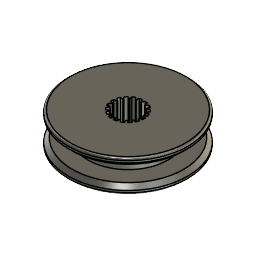
Spool60KGV0_v2 (Autodesk Fusion 360 design; units mm, degrees)
Autodesk Fusion 360 part; units mm, degrees
sketch "Sketch1" plane through (0, 0, 0) normal (0, 0, 1) x (1, 0, 0)
  line L0 (2.1718, 2.3549) -> (1.942, 2.5478)
  line L1 (2.1718, -2.3549) -> (2.7951, -2.7198)
  line L2 (-0.9579, 3.7805) -> (-0.9535, 3.0583)
  line L3 (1.942, -2.5478) -> (2.1718, -2.3549)
  line L4 (0.15, 3.2) -> (-0.15, 3.2)
  arc A0 (3.5568, -1.5998) -> (3.753, -1.0607) centre (0, 0) ccw
  line L5 (-0.15, 3.2) -> (-0.3929, 3.8802)
  arc A1 (3.753, 1.0607) -> (3.5568, 1.5998) centre (0, 0) ccw
  arc A2 (1.6963, -3.5118) -> (2.1931, -3.2249) centre (0, 0) ccw
  line L6 (2.7951, 2.7198) -> (2.1718, 2.3549)
  line L7 (-3.1253, -0.7034) -> (-3.753, -1.0607)
  arc A3 (-3.5568, 1.5998) -> (-3.753, 1.0607) centre (0, 0) ccw
  line L8 (-2.6963, 1.7299) -> (-2.8463, 1.4701)
  circle A4 centre (0, 0) radius 1.5
  line L9 (-3.1639, 2.2804) -> (-2.6963, 1.7299)
  line L10 (-3.1774, 0.408) -> (-3.8894, 0.2868)
  line L11 (-2.8463, 1.4701) -> (-3.5568, 1.5998)
  line L12 (-3.1253, 0.7034) -> (-3.1774, 0.408)
  line L13 (3.8894, 0.2868) -> (3.1774, 0.408)
  line L14 (3.1253, 0.7034) -> (3.753, 1.0607)
  arc A5 (-3.8894, 0.2868) -> (-3.8894, -0.2868) centre (0, 0) ccw
  line L15 (-2.1718, 2.3549) -> (-2.7951, 2.7198)
  line L16 (3.5568, 1.5998) -> (2.8463, 1.4701)
  line L17 (0.9535, -3.0583) -> (1.2354, -2.9557)
  line L18 (-1.942, 2.5478) -> (-2.1718, 2.3549)
  line L19 (-3.753, 1.0607) -> (-3.1253, 0.7034)
  line L20 (-2.1931, 3.2249) -> (-1.942, 2.5478)
  line L21 (3.1774, 0.408) -> (3.1253, 0.7034)
  line L22 (2.8463, 1.4701) -> (2.6963, 1.7299)
  line L23 (0.3929, 3.8802) -> (0.15, 3.2)
  line L24 (-3.1774, -0.408) -> (-3.1253, -0.7034)
  line L25 (-0.9535, 3.0583) -> (-1.2354, 2.9557)
  arc A6 (3.1639, 2.2804) -> (2.7951, 2.7198) centre (0, 0) ccw
  line L26 (-3.8894, -0.2868) -> (-3.1774, -0.408)
  line L27 (2.1931, -3.2249) -> (1.942, -2.5478)
  arc A7 (-2.7951, 2.7198) -> (-3.1639, 2.2804) centre (0, 0) ccw
  arc A8 (-0.3929, 3.8802) -> (-0.9579, 3.7805) centre (0, 0) ccw
  arc A9 (-1.6963, 3.5118) -> (-2.1931, 3.2249) centre (0, 0) ccw
  arc A10 (2.7951, -2.7198) -> (3.1639, -2.2804) centre (0, 0) ccw
  line L28 (2.6963, 1.7299) -> (3.1639, 2.2804)
  line L29 (1.2354, -2.9557) -> (1.6963, -3.5118)
  line L30 (-1.2354, 2.9557) -> (-1.6963, 3.5118)
  line L31 (0.9579, -3.7805) -> (0.9535, -3.0583)
  line L32 (3.1774, -0.408) -> (3.8894, -0.2868)
  line L33 (2.8463, -1.4701) -> (3.5568, -1.5998)
  line L34 (-3.5568, -1.5998) -> (-2.8463, -1.4701)
  line L35 (3.1639, -2.2804) -> (2.6963, -1.7299)
  arc A11 (2.1931, 3.2249) -> (1.6963, 3.5118) centre (0, 0) ccw
  line L36 (1.2354, 2.9557) -> (0.9535, 3.0583)
  line L37 (0.15, -3.2) -> (0.3929, -3.8802)
  line L38 (3.753, -1.0607) -> (3.1253, -0.7034)
  line L39 (1.6963, 3.5118) -> (1.2354, 2.9557)
  line L40 (-2.8463, -1.4701) -> (-2.6963, -1.7299)
  line L41 (1.942, 2.5478) -> (2.1931, 3.2249)
  line L42 (2.6963, -1.7299) -> (2.8463, -1.4701)
  line L43 (0.9535, 3.0583) -> (0.9579, 3.7805)
  arc A12 (0.3929, -3.8802) -> (0.9579, -3.7805) centre (0, 0) ccw
  line L44 (3.1253, -0.7034) -> (3.1774, -0.408)
  line L45 (-2.6963, -1.7299) -> (-3.1639, -2.2804)
  arc A13 (-2.1931, -3.2249) -> (-1.6963, -3.5118) centre (0, 0) ccw
  line L46 (-2.7951, -2.7198) -> (-2.1718, -2.3549)
  arc A14 (0.9579, 3.7805) -> (0.3929, 3.8802) centre (0, 0) ccw
  line L47 (-0.3929, -3.8802) -> (-0.15, -3.2)
  line L48 (-2.1718, -2.3549) -> (-1.942, -2.5478)
  line L49 (-1.6963, -3.5118) -> (-1.2354, -2.9557)
  line L50 (-1.2354, -2.9557) -> (-0.9535, -3.0583)
  line L51 (-0.9535, -3.0583) -> (-0.9579, -3.7805)
  arc A15 (-3.1639, -2.2804) -> (-2.7951, -2.7198) centre (0, 0) ccw
  arc A16 (-0.9579, -3.7805) -> (-0.3929, -3.8802) centre (0, 0) ccw
  line L52 (-0.15, -3.2) -> (0.15, -3.2)
  arc A17 (3.8894, -0.2868) -> (3.8894, 0.2868) centre (0, 0) ccw
  arc A18 (-3.753, -1.0607) -> (-3.5568, -1.5998) centre (0, 0) ccw
  line L53 (-1.942, -2.5478) -> (-2.1931, -3.2249)
  arc A19 (-3.8698, -1.0122) -> (-3.6151, -1.7121) centre (0, 0) ccw
  line L54 (-3.6151, -1.7121) -> (-2.8976, -1.5811)
  line L55 (-2.8976, -1.5811) -> (-2.8181, -1.7189)
  line L56 (-2.8181, -1.7189) -> (-3.2903, -2.2747)
  arc A20 (-3.2903, -2.2747) -> (-2.8115, -2.8453) centre (0, 0) ccw
  line L57 (-2.8115, -2.8453) -> (-2.1821, -2.4768)
  line L58 (-2.1821, -2.4768) -> (-2.0603, -2.5791)
  line L59 (-2.0603, -2.5791) -> (-2.3138, -3.2628)
  arc A21 (-2.3138, -3.2628) -> (-1.6688, -3.6353) centre (0, 0) ccw
  line L60 (-1.6688, -3.6353) -> (-1.2034, -3.0738)
  line L61 (-1.2034, -3.0738) -> (-1.0539, -3.1282)
  line L62 (-1.0539, -3.1282) -> (-1.0583, -3.8574)
  arc A22 (-1.0583, -3.8574) -> (-0.3248, -3.9868) centre (0, 0) ccw
  line L63 (-0.3248, -3.9868) -> (-0.0795, -3.3)
  line L64 (-0.0795, -3.3) -> (0.0795, -3.3)
  line L65 (0.0795, -3.3) -> (0.3248, -3.9868)
  arc A23 (0.3248, -3.9868) -> (1.0583, -3.8574) centre (0, 0) ccw
  line L66 (1.0583, -3.8574) -> (1.0539, -3.1282)
  line L67 (1.0539, -3.1282) -> (1.2034, -3.0738)
  line L68 (1.2034, -3.0738) -> (1.6688, -3.6353)
  arc A24 (1.6688, -3.6353) -> (2.3138, -3.2628) centre (0, 0) ccw
  line L69 (2.3138, -3.2628) -> (2.0603, -2.5791)
  line L70 (2.0603, -2.5791) -> (2.1821, -2.4768)
  line L71 (2.1821, -2.4768) -> (2.8115, -2.8453)
  arc A25 (2.8115, -2.8453) -> (3.2903, -2.2747) centre (0, 0) ccw
  line L72 (3.2903, -2.2747) -> (2.8181, -1.7189)
  line L73 (2.8181, -1.7189) -> (2.8976, -1.5811)
  line L74 (2.8976, -1.5811) -> (3.6151, -1.7121)
  arc A26 (3.6151, -1.7121) -> (3.8698, -1.0122) centre (0, 0) ccw
  line L75 (3.8698, -1.0122) -> (3.2361, -0.6514)
  line L76 (3.2361, -0.6514) -> (3.2637, -0.4947)
  line L77 (3.2637, -0.4947) -> (3.9826, -0.3724)
  arc A27 (3.9826, -0.3724) -> (3.9826, 0.3724) centre (0, 0) ccw
  line L78 (3.9826, 0.3724) -> (3.2637, 0.4947)
  line L79 (3.2637, 0.4947) -> (3.2361, 0.6514)
  line L80 (3.2361, 0.6514) -> (3.8698, 1.0122)
  arc A28 (3.8698, 1.0122) -> (3.6151, 1.7121) centre (0, 0) ccw
  line L81 (3.6151, 1.7121) -> (2.8976, 1.5811)
  line L82 (2.8976, 1.5811) -> (2.8181, 1.7189)
  line L83 (2.8181, 1.7189) -> (3.2903, 2.2747)
  arc A29 (3.2903, 2.2747) -> (2.8115, 2.8453) centre (0, 0) ccw
  line L84 (2.8115, 2.8453) -> (2.1821, 2.4768)
  line L85 (2.1821, 2.4768) -> (2.0603, 2.5791)
  line L86 (2.0603, 2.5791) -> (2.3138, 3.2628)
  arc A30 (2.3138, 3.2628) -> (1.6688, 3.6353) centre (0, 0) ccw
  line L87 (1.6688, 3.6353) -> (1.2034, 3.0738)
  line L88 (1.2034, 3.0738) -> (1.0539, 3.1282)
  line L89 (1.0539, 3.1282) -> (1.0583, 3.8574)
  arc A31 (1.0583, 3.8574) -> (0.3248, 3.9868) centre (0, 0) ccw
  line L90 (0.3248, 3.9868) -> (0.0795, 3.3)
  line L91 (0.0795, 3.3) -> (-0.0795, 3.3)
  line L92 (-0.0795, 3.3) -> (-0.3248, 3.9868)
  arc A32 (-0.3248, 3.9868) -> (-1.0583, 3.8574) centre (0, 0) ccw
  line L93 (-1.0583, 3.8574) -> (-1.0539, 3.1282)
  line L94 (-1.0539, 3.1282) -> (-1.2034, 3.0738)
  line L95 (-1.2034, 3.0738) -> (-1.6688, 3.6353)
  arc A33 (-1.6688, 3.6353) -> (-2.3138, 3.2628) centre (0, 0) ccw
  line L96 (-2.3138, 3.2628) -> (-2.0603, 2.5791)
  line L97 (-2.0603, 2.5791) -> (-2.1821, 2.4768)
  line L98 (-2.1821, 2.4768) -> (-2.8115, 2.8453)
  arc A34 (-2.8115, 2.8453) -> (-3.2903, 2.2747) centre (0, 0) ccw
  line L99 (-3.2903, 2.2747) -> (-2.8181, 1.7189)
  line L100 (-2.8181, 1.7189) -> (-2.8976, 1.5811)
  line L101 (-2.8976, 1.5811) -> (-3.6151, 1.7121)
  arc A35 (-3.6151, 1.7121) -> (-3.8698, 1.0122) centre (0, 0) ccw
  line L102 (-3.8698, 1.0122) -> (-3.2361, 0.6514)
  line L103 (-3.2361, 0.6514) -> (-3.2637, 0.4947)
  line L104 (-3.2637, 0.4947) -> (-3.9826, 0.3724)
  arc A36 (-3.9826, 0.3724) -> (-3.9826, -0.3724) centre (0, 0) ccw
  line L105 (-3.9826, -0.3724) -> (-3.2637, -0.4947)
  line L106 (-3.2637, -0.4947) -> (-3.2361, -0.6514)
  line L107 (-3.2361, -0.6514) -> (-3.8698, -1.0122)
  circle A37 centre (0, 0) radius 10
  circle A38 centre (0, 0) radius 15
  dimension "d1" = 0.1
  dimension "d2" = 20
  dimension "d3" = 30
  dimension "d6" = 3
  constraint concentric A0 A37
  constraint concentric A0 A38
  measures "d2" diameter of A37
  measures "d3" diameter of A38
  measures "d6" diameter of A4
extrude "Extrude1" add sketch "Sketch1" along normal blind 8 contours A37 | A38
extrude "Extrude2" add sketch "Sketch1" along normal blind 2 contours L0 L1 L2 L3 L4 A0 L5 A1 A2 L6 L7 A3 L8 L9 L10 L11 L12 L13 L14 A5 L15 L16 L17 L18 L19 L20 L21 L22 L23 L24 L25 A6 L26 L27 A7 A8 A9 A10 L28 L29 L30 L31 L32 L33 L34 L35 A11 L36 L37 L38 L39 L40 L41 L42 L43 A12 L44 L45 A13 L46 A14 L47 L48 L49 L50 L51 A15 A16 L52 A17 A18 L53 | A19 L54 L55 L56 A20 L57 L58 L59 A21 L60 L61 L62 A22 L63 L64 L65 A23 L66 L67 L68 A24 L69 L70 L71 A25 L72 L73 L74 A26 L75 L76 L77 A27 L78 L79 L80 A28 L81 L82 L83 A29 L84 L85 L86 A30 L87 L88 L89 A31 L90 L91 L92 A32 L93 L94 L95 A33 L96 L97 L98 A34 L99 L100 L101 A35 L102 L103 L104 A36 L105 L106 L107
extrude "Extrude3" cut sketch "Sketch1" along normal blind 4 from surface at 2 contours A38
fillet "Fillet1" radius 0.5 2 edges at (-13.9849, -5.4242, 0) (-13.9849, -5.4242, 8)
chamfer "Chamfer1" distance 1 angle 45 2 edges at (-13.9849, 5.4242, 2) (-13.9849, -5.4242, 6) tangent chain off
hole "Hole1" at (-5.3208, 8.9613, 2) direction (0, 0, -1) diameter 3 depth 3 tip angle 180
fillet "Fillet2" radius 0.85 2 edges at (-4.555, 7.6715, 2) (-5.1054, 8.5985, 2)
